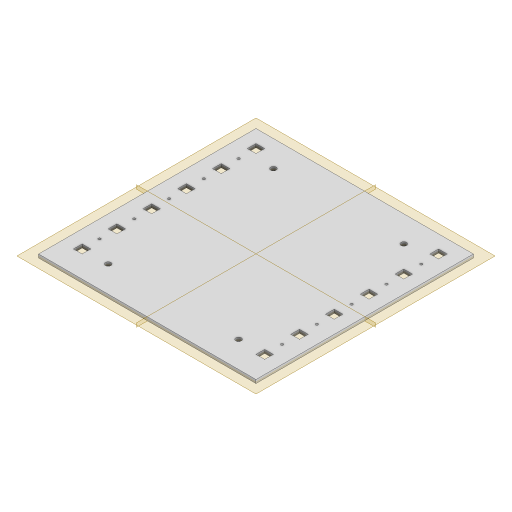
# Autodesk Inventor part: Основание подъёмника
Saved by Autodesk Inventor 2023.2 (Build 272271030, 271C)
## iProperties
Created: 2025-03-19
Part Number: Основание подъёмника
Material: Типовые
Document SubType Name: Modeling
Designer: Коноваленко
Density: 1 g/cm^3
Appearance: По умолчанию
Author: Коноваленко
Autodesk Inventor part; units mm, degrees
sketch "Эскиз1" plane through (0, 0, 0) normal (0, 1, 0) x (-1, 0, 0)
  line L0 (125, 125) -> (-125, 125)
  line L1 (-125, 125) -> (-125, -125)
  line L2 (-125, -125) -> (125, -125)
  line L3 (125, -125) -> (125, 125)
  line L4 (125, 125) -> (-125, -125) construction
  line L5 (-125, 125) -> (125, -125) construction
  point P0 (0, 0)
  dimension "d0" = 250
  dimension "d1" = 250
  constraints: 12 end point, 2 midpoint, 2 parallel, 1 horizontal, 1 perpendicular
  measures "d0" distance of L0.end L1.end
  measures "d1" distance of L1.end L2.end
extrude "Выдавливание1" add sketch "Эскиз1" along normal mid plane 4
sketch "Эскиз2" plane through (0, -2, 0) normal (0, -1, 0) x (1, 0, 0)
  line L0 (-110, 100) -> (-100, 100) projected
  line L1 (-110, 90) -> (-110, 100) projected
  line L2 (-100, 90) -> (-110, 90) projected
  line L3 (-100, 100) -> (-100, 90) projected
  line L4 (-110, 20) -> (-100, 20) projected
  line L5 (-100, 10) -> (-110, 10) projected
  line L6 (-110, 10) -> (-110, 20) projected
  line L7 (-100, 20) -> (-100, 10) projected
  line L8 (-100, -20) -> (-100, -30) projected
  line L9 (-100, -30) -> (-110, -30) projected
  line L10 (-110, -30) -> (-110, -20) projected
  line L11 (-110, -20) -> (-100, -20) projected
  line L12 (-100, -60) -> (-100, -70) projected
  line L13 (-100, -70) -> (-110, -70) projected
  line L14 (-110, -70) -> (-110, -60) projected
  line L15 (-110, -60) -> (-100, -60) projected
  line L16 (-100, -100) -> (-100, -110) projected
  line L17 (-100, -110) -> (-110, -110) projected
  line L18 (-110, -100) -> (-100, -100) projected
  line L19 (-110, -110) -> (-110, -100) projected
  line L20 (110, -110) -> (110, -100) projected
  line L21 (100, -110) -> (110, -110) projected
  line L22 (110, -100) -> (100, -100) projected
  line L23 (100, -100) -> (100, -110) projected
  line L24 (100, -60) -> (100, -70) projected
  line L25 (100, -70) -> (110, -70) projected
  line L26 (110, -70) -> (110, -60) projected
  line L27 (110, -60) -> (100, -60) projected
  line L28 (100, -30) -> (110, -30) projected
  line L29 (110, -30) -> (110, -20) projected
  line L30 (110, -20) -> (100, -20) projected
  line L31 (100, -20) -> (100, -30) projected
  line L32 (100, 10) -> (110, 10) projected
  line L33 (110, 10) -> (110, 20) projected
  line L34 (100, 20) -> (100, 10) projected
  line L35 (110, 20) -> (100, 20) projected
  line L36 (100, 90) -> (110, 90) projected
  line L37 (110, 100) -> (100, 100) projected
  line L38 (110, 90) -> (110, 100) projected
  line L39 (100, 100) -> (100, 90) projected
  line L40 (-110, 50) -> (-110, 55) projected
  line L41 (-110, 55) -> (-110, 60) projected
  line L42 (-110, 60) -> (-100, 60) projected
  line L43 (-100, 60) -> (-100, 55) projected
  line L44 (-100, 55) -> (-100, 50) projected
  line L45 (-100, 50) -> (-110, 50) projected
  line L46 (110, 55) -> (110, 60) projected
  line L47 (110, 60) -> (100, 60) projected
  line L48 (110, 50) -> (110, 55) projected
  line L49 (100, 50) -> (110, 50) projected
  line L50 (100, 55) -> (100, 50) projected
  line L51 (100, 60) -> (100, 55) projected
  circle A0 centre (-105, -85) radius 2 construction
  circle A1 centre (-105, -45) radius 2 construction
  circle A2 centre (-105, -5) radius 2 construction
  circle A3 centre (-105, 35) radius 2 construction
  circle A4 centre (-105, 75) radius 2 construction
  circle A5 centre (105, 75) radius 2 construction
  circle A6 centre (105, 35) radius 2 construction
  circle A7 centre (105, -5) radius 2 construction
  circle A8 centre (105, -45) radius 2 construction
  circle A9 centre (105, -85) radius 2 construction
  circle A10 centre (-105, 75) radius 1.45
  circle A11 centre (-105, 35) radius 1.45
  circle A12 centre (-105, -5) radius 1.45
  circle A13 centre (-105, -45) radius 1.45
  circle A14 centre (-105, -85) radius 1.45
  circle A15 centre (105, 75) radius 1.45
  circle A16 centre (105, 35) radius 1.45
  circle A17 centre (105, -5) radius 1.45
  circle A18 centre (105, -45) radius 1.45
  circle A19 centre (105, -85) radius 1.45
  point P0 (0, 0)
  dimension "d18" = 2.9
  dimension "d21" = 40
  dimension "d24" = 210
  constraints: 10 centre point, 1 horizontal, 1 vertical, 18 other
  measures "d18" diameter of A10
  measures "d21" distance of A4.centre A11.centre
  measures "d24" distance of A4.centre A15.centre
extrude "Выдавливание2" cut sketch "Эскиз2" against normal up to surface (4 mm away)
sketch "Эскиз3" plane through (0, -2, 0) normal (0, -1, 0) x (1, 0, 0)
  circle A0 centre (75, -95) radius 3.15
  line L0 (125, -125) -> (125, 125) projected
  line L1 (-125, -125) -> (125, -125) projected
  line L2 (0, -76.118) -> (0, 76.118) construction
  line L3 (24.9561, 0) -> (-24.9561, 0) construction
  circle A1 centre (-75, -95) radius 3.15
  line L4 (-24.9561, 0) -> (24.9561, 0) construction
  circle A2 centre (75, 95) radius 3.15
  circle A3 centre (-75, 95) radius 3.15
  point P0 (0, 0)
  point P1 (0, 0)
  dimension "d10" = 6.3
  dimension "d14" = 50
  dimension "d15" = 30
  constraints: 6 end point, 5 symmetric about line, 4 centre point, 2 midpoint, 1 coincident, 1 horizontal, 1 vertical, 3 other
  measures "d10" diameter of A0
  measures "d14" distance from line of L0 A0.centre
  measures "d15" distance from line of L1 A0.centre
extrude "Выдавливание3" cut sketch "Эскиз3" against normal up to surface (4 mm away)
